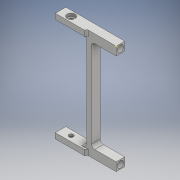
# Autodesk Inventor part: mtv_backHolder(4_30)
Saved by Autodesk Inventor 2018 (Build 220112000, 112)
## iProperties
Created: 2019-04-30
Part Number: mtv_backHolder(4_30)
Material: Generic
Document SubType Name: Modeling
Designer: Aditya Kendre
Density: 1 g/cm^3
Appearance: Default
Author: Aditya Kendre
## iProperties of the stored document mtv_backHolder(4_30)_3DPrint.ipt
Created: 2019-04-30
Part Number: mtv_backHolder(4_30)_3DPrint
Material: Generic
Document SubType Name: Modeling
Designer: Aditya Kendre
Density: 1 g/cm^3
Appearance: Default
Author: Aditya Kendre
Autodesk Inventor part; units mm, degrees
ref_plane "YZ Plane" through (0, 0, 0) normal (1, 0, 0) x (0, 1, 0)
ref_plane "XZ Plane" through (0, 0, 0) normal (0, 1, 0) x (-1, 0, 0)
ref_plane "XY Plane" through (0, 0, 0) normal (0, 0, 1) x (1, 0, 0)
sketch "Sketch1" plane through (0, 0, 0) normal (1, 0, 0) x (0, 1, 0)
  line L0 (0, 0) -> (8.763, 0)
  line L1 (8.763, 0) -> (8.763, -5.5118)
  line L2 (8.763, -5.5118) -> (0, -5.5118)
  line L3 (0, -5.5118) -> (0, 0)
  line L4 (1.5875, -3.9243) -> (7.1755, -3.9243)
  line L5 (7.1755, -3.9243) -> (7.1755, -1.5875)
  line L6 (7.1755, -1.5875) -> (1.5875, -1.5875)
  line L7 (1.5875, -1.5875) -> (1.5875, -3.9243)
  line L8 (1.5875, -3.9243) -> (7.1755, -1.5875) construction
  line L9 (7.1755, -3.9243) -> (1.5875, -1.5875) construction
  line L10 (0, -105.512) -> (8.763, -105.512)
  line L11 (8.763, -105.512) -> (8.763, -111.0238)
  line L12 (8.763, -111.0238) -> (0, -111.0238)
  line L13 (0, -111.0238) -> (0, -105.512)
  line L14 (1.5875, -109.4363) -> (7.1755, -109.4363)
  line L15 (7.1755, -109.4363) -> (7.1755, -107.0995)
  line L16 (7.1755, -107.0995) -> (1.5875, -107.0995)
  line L17 (1.5875, -107.0995) -> (1.5875, -109.4363)
  line L18 (1.5875, -109.4363) -> (7.1755, -107.0995) construction
  line L19 (7.1755, -109.4363) -> (1.5875, -107.0995) construction
  point P0 (4.3815, -2.7559)
  point P1 (4.3815, -108.2679)
  dimension "d0" = 8.763
  dimension "d1" = 5.5118
  dimension "d4" = 5.588
  dimension "d5" = 2.3368
  dimension "d6" = 8.763
  dimension "d7" = 5.5118
  dimension "d8" = 5.588
  dimension "d9" = 2.3368
  constraints: 40 end point, 8 parallel, 4 horizontal, 4 midpoint, 4 perpendicular
  measures "d0" distance of L1.end L2.end
  measures "d1" distance of L0.end L1.end
  measures "d4" distance of L6.end L5.end
  measures "d5" distance of L5.end L4.end
  measures "d6" distance of L11.end L12.end
  measures "d7" distance of L10.end L11.end
  measures "d8" distance of L16.end L15.end
  measures "d9" distance of L15.end L14.end
extrude "Extrusion1" add sketch "Sketch1" against normal blind 30
sketch "Sketch2" plane through (0, 0, -111.0238) normal (0, 0, -1) x (-1, 0, 0)
  line L0 (0, 8.763) -> (30, 8.763) projected
  line L1 (0, 0) -> (30, 0) projected
  line L2 (30, 8.763) -> (25, 8.763)
  line L3 (25, 8.763) -> (25, 0)
  line L4 (25, 0) -> (30, 0)
  line L5 (30, 0) -> (30, 8.763)
  dimension "d12" = 5
  constraints: 8 end point, 2 parallel, 1 horizontal, 1 perpendicular, 1 point on line
  measures "d12" distance of L4.end L3.end
extrude "Extrusion2" add sketch "Sketch2" against normal blind 111
sketch "Sketch3" plane through (-30, 0, 0) normal (-1, 0, 0) x (0, 0, 1)
  line L0 (-111.0238, 8.763) -> (-111.0238, 0) projected
  line L1 (-111.0238, 8.763) -> (-105.512, 8.763)
  line L2 (-105.512, 8.763) -> (-105.512, -2)
  line L3 (-105.512, -2) -> (-111.0238, -2)
  line L4 (-111.0238, -2) -> (-111.0238, 8.763)
  line L5 (0, 8.763) -> (-5.5118, 8.763) projected
  line L6 (0, 8.763) -> (-5.5118, 8.763)
  line L7 (-5.5118, 8.763) -> (-5.5118, -2)
  line L8 (-5.5118, -2) -> (0, -2)
  line L9 (0, -2) -> (0, 8.763)
  point P0 (0, 0)
  dimension "d15" = 10.763
  dimension "d16" = 10.763
  constraints: 16 end point, 4 parallel, 2 horizontal, 2 perpendicular
  measures "d15" distance of L1.end L2.end
  measures "d16" distance of L7.end L6.end
extrude "Extrusion3" add sketch "Sketch3" along normal blind 30
fillet "Fillet1" radius 2 2 edges at (-30, 0, -2.7559) (-30, 0, -108.2679)
fillet "Fillet2" radius 5 4 edges at (-30, 4.3815, -5.5118) (-25, 4.3815, -105.512) (-25, 4.3815, -5.5118) (-30, 4.3815, -105.512)
sketch "Sketch4" plane through (0, 0, 0) normal (0, 0, 1) x (1, 0, 0)
  line L0 (-30, -2) -> (-60, -2) construction
  line L1 (-60, 8.763) -> (-49.237, 8.763) construction
  line L2 (-49.237, 8.763) -> (-49.237, -2) construction
  line L3 (-49.237, -2) -> (-60, -2) construction
  line L4 (-60, -2) -> (-60, 8.763) construction
  circle A0 centre (-49.237, 3.3815) radius 4.05
  point P0 (0, 0)
  dimension "d21" = 10.763
  dimension "d22" = 8.1
  constraints: 8 end point, 2 parallel, 1 centre point, 1 horizontal, 1 midpoint, 1 perpendicular, 1 point on line
  measures "d21" distance of L2.end L3.end
  measures "d22" diameter of A0
extrude "Extrusion4" cut sketch "Sketch4" against normal blind 114.75
sketch "Sketch5" plane through (-60, -2, -105.512) normal (0, 0, 1) x (1, 0, 0)
  circle A0 centre (10.763, 5.3815) radius 4.05 projected
  circle A1 centre (10.763, 5.3815) radius 4.05
  point P0 (60, 2)
  constraints: 1 centre point, 1 coincident
extrude "Extrusion5" add sketch "Sketch5" against normal blind 2.412
sketch "Sketch6" plane through (-60, -2, -5.5118) normal (0, 0, -1) x (-1, 0, 0)
  circle A0 centre (-10.763, 5.3815) radius 4.05 projected
  circle A1 centre (-10.763, 5.3815) radius 4.05
  point P0 (-60, 2)
  constraints: 1 centre point, 1 coincident
extrude "Extrusion6" add sketch "Sketch6" against normal blind 2.412
sketch "Sketch7" plane through (-49.237, 3.3815, -107.924) normal (0, 0, -1) x (-1, 0, 0)
  circle A0 centre (0, 0) radius 2.25
  point P0 (-49.237, -3.3815)
  dimension "d29" = 4.5
  constraints: 1 centre point
  measures "d29" diameter of A0
extrude "Extrusion7" cut sketch "Sketch7" against normal blind 115
fillet "Fillet3" radius 0.5 8 edges at (0, 7.1755, -108.2679) (0, 4.3815, -107.0995) (0, 4.3815, -109.4363) (0, 1.5875, -108.2679) (0, 7.1755, -2.7559) (0, 4.3815, -1.5875) (0, 4.3815, -3.9243) (0, 1.5875, -2.7559)
sketch "Sketch8" plane through (0, 0, 0) normal (1, 0, 0) x (0, 0, -1)
  point P0 (0, 0)
sketch "Sketch9" plane through (0, 0, 0) normal (1, 0, 0) x (0, 0, -1)
  line L0 (0, -2) -> (0, 8.763) projected
  line L1 (5.5118, 0) -> (10.5118, 0) projected
  line L2 (0, 8.763) -> (8.763, 8.763)
  line L3 (8.763, 8.763) -> (8.763, 0)
  line L4 (8.763, 0) -> (0, 0)
  line L5 (0, 0) -> (0, 8.763)
  line L6 (105.512, 8.763) -> (111.0238, 8.763) projected
  line L7 (111.0238, 8.763) -> (102.2608, 8.763)
  line L8 (102.2608, 8.763) -> (102.2608, 0)
  line L9 (102.2608, 0) -> (111.0238, 0)
  line L10 (111.0238, 0) -> (111.0238, 8.763)
  dimension "d33" = 8.763
  dimension "d34" = 8.763
  constraints: 16 end point, 4 parallel, 2 horizontal, 2 perpendicular, 1 point on line
  measures "d33" distance of L3.end L4.end
  measures "d34" distance of L9.end L8.end
extrude "Extrusion8" add sketch "Sketch9" against normal blind 29.5
sketch "Sketch10" plane through (0, 0, 0) normal (1, 0, 0) x (0, 0, -1)
  line L0 (0, 0) -> (0, 8.763) construction
  line L1 (8.763, 0) -> (10.5118, 0) construction
  line L2 (0, 8.763) -> (8.763, 0) construction
  line L3 (8.763, 0) -> (8.763, 8.763) construction
  line L4 (0, 0) -> (0, -2) construction
  line L5 (8.763, 8.763) -> (0, 0) construction
  line L6 (111.0238, 8.763) -> (111.0238, -2) construction
  line L7 (100.512, 0) -> (102.2608, 0) construction
  line L8 (111.0238, 8.763) -> (102.2608, 0) construction
  line L9 (102.2608, 0) -> (102.2608, 8.763) construction
  line L10 (111.0238, 0) -> (102.2608, 0) construction
  line L11 (102.2608, 8.763) -> (111.0238, 0) construction
  circle A0 centre (106.6423, 4.3815) radius 3.25
  circle A1 centre (4.3815, 4.3815) radius 3.25
  dimension "d37" = 6.5
  dimension "d38" = 6.5
  constraints: 12 end point, 4 perpendicular, 2 centre point, 2 midpoint
  measures "d37" diameter of A0
  measures "d38" diameter of A1
extrude "Extrusion9" cut sketch "Sketch10" against normal blind 24.75
fillet "Fillet4" radius 3.25 2 edges at (-24.6842, 4.3815, -8.763) (-24.6842, 4.3815, -102.2608)
body "Solid1"
